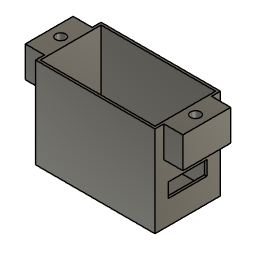
Servo Box v3 (Autodesk Fusion 360 design; units mm, degrees)
Autodesk Fusion 360 part; units mm, degrees
sketch "Sketch1" plane through (0, 0, 0) normal (0, 0, 1) x (1, 0, 0)
  line L0 (-25, -11.4) -> (-25, 2.3)
  line L1 (-25, 2.3) -> (0, 2.3)
  line L2 (0, 2.3) -> (0, -11.4)
  line L3 (0, -11.4) -> (-25, -11.4)
  dimension "d1" = 13.7
  dimension "d2" = 25
  constraint perpendicular L0 L1
  constraint perpendicular L1 L2
  constraint perpendicular L0 L3
  measures "d1" distance of L0.start L0.end
  measures "d2" distance of L0.end L1.end
extrude "Extrude1" add sketch "Sketch1" along normal blind 19
shell "Shell1" thickness 0.5 removed faces 1 at (-8.3333, -6.8333, 19)
sketch "Sketch2" plane through (0, 0, 0) normal (1, 0, 0) x (0, 1, 0)
  line L0 (-11.4, 0) -> (2.3, 0)
  line L1 (2.3, 0) -> (2.3, 19)
  line L2 (2.3, 19) -> (-11.4, 19)
  line L3 (-11.4, 19) -> (-11.4, 0)
  line L4 (-8.6, 8) -> (-0.5, 8)
  line L5 (-0.5, 8) -> (-0.5, 5)
  line L6 (-0.5, 5) -> (-8.6, 5)
  line L7 (-8.6, 5) -> (-8.6, 8)
  dimension "d6" = 5
  dimension "d7" = 8.1
  dimension "d8" = 2.8
  dimension "d9" = 2.8
  constraint horizontal L4
  constraint vertical L5
  constraint horizontal L6
  constraint vertical L7
  measures "d6" distance of L0 L6
  measures "d7" distance of L4.start L4.end
  measures "d8" distance of L3 L7
  measures "d9" distance of L1 L5
extrude "Extrude2" cut sketch "Sketch2" along normal mid plane 6 contours L4 L5 L6 L7
sketch "Sketch3" plane through (0, 0, 0) normal (1, 0, 0) x (0, 1, 0)
  line L0 (-0.5, 8) -> (-0.5, 5)
  line L1 (-0.5, 5) -> (-8.6, 5)
  line L2 (-8.6, 5) -> (-8.6, 8)
  line L3 (-8.6, 8) -> (-0.5, 8)
  line L4 (-11.4, 0) -> (2.3, 0)
  line L5 (2.3, 0) -> (2.3, 19)
  line L6 (2.3, 19) -> (-11.4, 19)
  line L7 (-11.4, 19) -> (-11.4, 0)
  line L8 (-9.55, 19) -> (0.45, 19)
  line L9 (0.45, 19) -> (0.45, 12.5)
  line L10 (0.45, 12.5) -> (-9.55, 12.5)
  line L11 (-9.55, 12.5) -> (-9.55, 19)
  dimension "d19" = 10
  dimension "d20" = 1.85
  dimension "d23" = 6.5
  constraint horizontal L8
  constraint vertical L9
  constraint horizontal L10
  constraint vertical L11
  constraint coincident L6 L8.start
  measures "d19" distance of L9.end L10.end
  measures "d20" distance of L5 L9
  measures "d23" distance of L8.start L10.end
extrude "Extrude3" add sketch "Sketch3" along normal blind 4 contours L6 L8 L9 L10 L11
sketch "Sketch4" plane through (0, 0, 19) normal (0, 0, 1) x (-1, 0, 0)
  line L0 (0.5, 10.9) -> (24.5, 10.9)
  line L1 (24.5, 10.9) -> (24.5, -1.8)
  line L2 (24.5, -1.8) -> (0.5, -1.8)
  line L3 (0.5, -1.8) -> (0.5, 10.9)
  line L4 (0, 11.4) -> (0, 9.55)
  line L5 (0, 9.55) -> (-4, 9.55)
  line L6 (-4, 9.55) -> (-4, -0.45)
  line L7 (-4, -0.45) -> (0, -0.45)
  line L8 (0, -0.45) -> (0, -2.3)
  line L9 (0, -2.3) -> (25, -2.3)
  line L10 (25, -2.3) -> (25, 11.4)
  line L11 (25, 11.4) -> (0, 11.4)
  circle A0 centre (-1.65, 4.55) radius 1.025
  dimension "d16" = 2.05
  dimension "d32" = 5
  dimension "d33" = 2.15
  measures "d16" diameter of A0
  measures "d32" distance of L7 A0.centre
  measures "d33" distance of L3 A0.centre
extrude "Extrude4" cut sketch "Sketch4" against normal blind 5.5 contours A0
sketch "Sketch6" plane through (-25, 0, 0) normal (-1, 0, 0) x (0, -1, 0)
  line L0 (-2.3, 0) -> (11.4, 0)
  line L1 (11.4, 0) -> (11.4, 19)
  line L2 (11.4, 19) -> (-2.3, 19)
  line L3 (-2.3, 19) -> (-2.3, 0)
  line L4 (-0.45, 19) -> (9.55, 19)
  line L5 (9.55, 19) -> (9.55, 12.5)
  line L6 (9.55, 12.5) -> (-0.45, 12.5)
  line L7 (-0.45, 12.5) -> (-0.45, 19)
  dimension "d27" = 1.85
  dimension "d28" = 10
  dimension "d29" = 6.5
  constraint horizontal L4
  constraint vertical L5
  constraint horizontal L6
  constraint vertical L7
  constraint coincident L2 L4.start
  measures "d27" distance of L1 L5
  measures "d28" distance of L5.end L6.end
  measures "d29" distance of L4.start L6.end
extrude "Extrude5" add sketch "Sketch6" along normal blind 4 contours L2 L4 L5 L6 L7
sketch "Sketch7" plane through (0, 0, 19) normal (0, 0, 1) x (-1, 0, 0)
  circle A0 centre (-1.65, 4.55) radius 1.025
  line L0 (0.5, 10.9) -> (24.5, 10.9)
  line L1 (24.5, 10.9) -> (24.5, -1.8)
  line L2 (24.5, -1.8) -> (0.5, -1.8)
  line L3 (0.5, -1.8) -> (0.5, 10.9)
  line L4 (0, 11.4) -> (0, 9.55)
  line L5 (0, 9.55) -> (-4, 9.55)
  line L6 (-4, 9.55) -> (-4, -0.45)
  line L7 (-4, -0.45) -> (0, -0.45)
  line L8 (0, -0.45) -> (0, -2.3)
  line L9 (0, -2.3) -> (25, -2.3)
  line L10 (25, -2.3) -> (25, -0.45)
  line L11 (25, -0.45) -> (29, -0.45)
  line L12 (29, -0.45) -> (29, 9.55)
  line L13 (29, 9.55) -> (25, 9.55)
  line L14 (25, 9.55) -> (25, 11.4)
  line L15 (25, 11.4) -> (0, 11.4)
  circle A1 centre (26.6, 4.55) radius 1.025
  dimension "d34" = 2.05
  dimension "d35" = 2.1
  dimension "d36" = 5
  measures "d34" diameter of A1
  measures "d35" distance of L1 A1.centre
  measures "d36" distance of L11 A1.centre
extrude "Extrude6" cut sketch "Sketch7" against normal blind 5.5 contours A1
